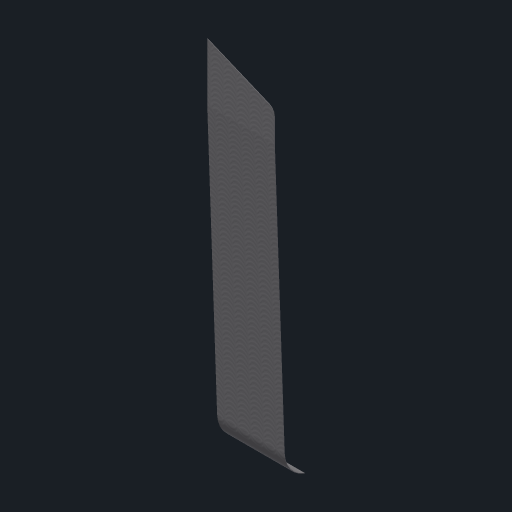
# Autodesk Inventor part: CHAPA_4_v2
Saved by Autodesk Inventor 2024.3 (Build 283343000, 343)
## iProperties
Created: 2024-06-30
Part Number: CHAPA_4_v2
Material: Steel, Mild, Welded
Document SubType Name: Sheet Metal
Designer: Niler
Density: 7.85 g/cm^3
Sheet Metal Rule: Default_mm
Appearance: Weld - Steel Mild
Author: Niler
Autodesk Inventor part; units mm, degrees
ref_plane "YZ Plane" through (0, 0, 0) normal (1, 0, 0) x (0, 1, 0)
ref_plane "XZ Plane" through (0, 0, 0) normal (0, 1, 0) x (-1, 0, 0)
ref_plane "XY Plane" through (0, 0, 0) normal (0, 0, 1) x (1, 0, 0)
sketch "Sketch1" plane through (0, 0, 0) normal (0, 0, 1) x (1, 0, 0)
  line L0 (0, 0) -> (0, 84)
  circle A0 centre (-30, 84) radius 30
  line L1 (-18.4615, 111.6923) -> (-233.4459, 201.2697)
  line L2 (-233.4459, 201.2697) -> (-233.4459, 0)
  line L3 (-233.4459, 0) -> (0, 0)
  dimension "d0" = 84
  dimension "d1" = 60
  dimension "d2" = 112.62
  dimension "d3" = 232.9
  measures "d0" distance of L0.start L0.end
  measures "d1" diameter of A0
  measures "d2" angle of L0 L1
  measures "d3" distance of L1.start L1.end
extrude "Plate1" add sketch "Sketch1" along normal blind 1.5
sketch "Sketch2" plane through (-233.4459, 0.0542, 0.001) normal (0, -0.0361205, 0.9993474) x (1, 0, 0)
  line L0 (233.4459, 0) -> (0, 0)
  line L1 (0, 0) -> (0, -948)
  line L2 (0, -948) -> (233.4459, -948)
  line L3 (233.4459, -948) -> (233.4459, 0)
  constraints: 6 end point, 1 horizontal, 1 perpendicular, 1 vertical
edge flange "Flange1" height 948 angle 2.07 thickness 1.5 bend radius 1 thickness toward (0, -0.0361205, 0.9993474) relief straight relief width 1.5 relief depth 0.75 edges at (-116.7229, 0, 0) wall of the first edge with corners at (0, 0.0542, 0.001) (-233.4459, 0.0542, 0.001) (-233.4459, -947.3272, -34.2412) (0, -947.3272, -34.2412)
bend "Bend1"
corner "Corner1"
sketch "Sketch3" plane through (-233.4459, -1046.604, -122.3369) normal (0, -0.9879599, 0.1547104) x (1, 0, 0)
  line L0 (233.4459, 0) -> (0, 0)
  line L1 (0, 0) -> (0, -12.7387)
  line L2 (0, -12.7387) -> (233.4459, -12.7387)
  line L3 (233.4459, -12.7387) -> (233.4459, 0)
  constraints: 6 end point, 1 horizontal, 1 perpendicular, 1 vertical
edge flange "Flange2" height 100 angle 79.03 thickness 1.5 bend radius 104.3 thickness toward (0, -0.9879599, 0.1547104) relief straight relief width 1.5 relief depth 0.75 edges at (-116.7229, -947.3272, -34.2412) wall of the first edge with corners at (0, -1046.604, -122.3369) (-233.4459, -1046.604, -122.3369) (-233.4459, -1048.5749, -134.9222) (0, -1048.5749, -134.9222)
bend "Bend2"
corner "Corner2"
sketch "Sketch4" plane through (0, -1050.0568, -134.6901) normal (1, 0, 0) x (0, -0.1547104, -0.9879599)
  line L0 (-12.7387, 1.5) -> (-12.7387, 0) projected
  arc A0 (-115.1328, 85.9522) -> (-12.7387, 1.5) centre (-12.7387, 105.8) ccw projected
  line L1 (-115.1328, 85.9522) -> (-116.6054, 85.6668) projected
  arc A1 (-116.6054, 85.6668) -> (-12.7387, 0) centre (-12.7387, 105.8) ccw projected
  line L2 (-31.7292, 3.2434) -> (-32.1983, 1.805)
  line L3 (-12.7387, 1.5) -> (-12.7387, 0) projected
  line L4 (-12.7387, 0) -> (0, 0) projected
  line L5 (0, 1.5) -> (0, 0) projected
  line L6 (0, 1.5) -> (-12.7387, 1.5) projected
  point P0 (-295.5231, 1016.576)
  constraints: 2 end point, 2 point on circle
extrude "Extrusion1" cut sketch "Sketch4" against normal through all contours L6 L5 L4 L0 | L0 A1 L2 A0
equation "\"d4\" = Thickness"
equation "\"d5\" = BendReliefWidth"
equation "\"d6\" = BendReliefDepth"
equation "\"d7\" = MinimumRemnant"
equation "\"d8\" = TransitionRadius"
equation "\"d12\" = CornerReliefSize"
equation "\"d13\" = GapSize"
equation "\"d14\" = JacobiRadiusSize"
equation "\"d15\" = BendReliefWidth"
equation "\"d16\" = BendReliefDepth"
equation "\"d17\" = MinimumRemnant"
equation "\"d18\" = TransitionRadius"
equation "\"d22\" = CornerReliefSize"
equation "\"d23\" = GapSize"
equation "\"d24\" = JacobiRadiusSize"
equation "\"BendRadius\" = Thickness"
equation "\"BendReliefWidth\" = Thickness"
equation "\"BendReliefDepth\" = 0.5 * Thickness"
equation "\"CornerReliefSize\" = 4 * Thickness"
equation "\"MinimumRemnant\" = 2 * Thickness"
equation "\"TransitionRadius\" = BendRadius"
equation "\"JacobiRadiusSize\" = BendRadius"
equation "\"GapSize\" = Thickness"
equation "\"Thickness\" = 1.5"
body "Solid1"
